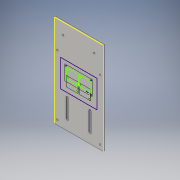
# Autodesk Inventor part: Part2
Saved by Autodesk Inventor 2016 (Build 200138000, 138)
## iProperties
Created: 2015-10-15
Part Number: Part2
Material: Generic
Document SubType Name: Modeling
Designer: hozhu
Density: 1 g/cm^3
Appearance: Default
Author: hozhu
Autodesk Inventor part; units mm, degrees
ref_plane "YZ Plane" through (0, 0, 0) normal (1, 0, 0) x (0, 1, 0)
ref_plane "XZ Plane" through (0, 0, 0) normal (0, 1, 0) x (-1, 0, 0)
ref_plane "XY Plane" through (0, 0, 0) normal (0, 0, 1) x (1, 0, 0)
sketch "Sketch1" plane through (0, 0, 0) normal (0, 0, 1) x (1, 0, 0)
  line L0 (-68.58, -128.7145) -> (68.58, -128.7145)
  line L1 (68.58, -128.7145) -> (68.58, 128.7145)
  line L2 (68.58, 128.7145) -> (-68.58, 128.7145)
  line L3 (-68.58, 128.7145) -> (-68.58, -128.7145)
  line L4 (-68.58, -128.7145) -> (68.58, 128.7145) construction
  line L5 (68.58, -128.7145) -> (-68.58, 128.7145) construction
  point P0 (0, 0)
  dimension "d0" = 137.16
  dimension "d1" = 257.429
  constraints: 12 end point, 2 midpoint, 2 parallel, 1 horizontal, 1 perpendicular
  measures "d0" distance of L1.end L2.end
  measures "d1" distance of L2.end L0.start
extrude "Extrusion1" add sketch "Sketch1" against normal blind 3.175
sketch "Sketch2" plane through (0, 0, 0) normal (0, 0, 1) x (1, 0, 0)
  circle A0 centre (-59.69, 52.5145) radius 2.0955
  line L0 (-68.58, 128.7145) -> (-68.58, -128.7145) projected
  line L1 (-68.58, 128.7145) -> (68.58, 128.7145) projected
  circle A1 centre (59.69, 52.5145) radius 2.0955
  line L2 (68.58, -128.7145) -> (68.58, 128.7145) projected
  circle A2 centre (-59.69, -116.0145) radius 2.0955
  circle A3 centre (59.69, -116.0145) radius 2.0955
  line L3 (-68.58, -128.7145) -> (68.58, -128.7145) projected
  point P0 (0, 0)
  dimension "d4" = 8.89
  dimension "d5" = 76.2
  dimension "d6" = 76.2
  dimension "d7" = 8.89
  dimension "d8" = 4.191
  dimension "d9" = 12.7
  dimension "d10" = 8.89
  dimension "d11" = 8.89
  dimension "d12" = 12.7
  dimension "d13" = 4.191
  dimension "d21" = 4.191
  dimension "d22" = 4.191
  constraints: 4 centre point
  measures "d4" distance from line of L0 A0.centre
  measures "d5" distance from line of L1 A0.centre
  measures "d6" distance from line of L1 A1.centre
  measures "d7" distance from line of A1.centre L2
  measures "d8" diameter of A1
  measures "d9" distance from line of L3 A2.centre
  measures "d10" distance from line of L0 A2.centre
  measures "d11" distance from line of L2 A3.centre
  measures "d12" distance from line of L3 A3.centre
  measures "d13" diameter of A0
  measures "d21" diameter of A2
  measures "d22" diameter of A3
hole "Hole1" at (-59.69, 52.5145, 0) at (59.69, 52.5145, 0) at (-59.69, -116.0145, 0) at (59.69, -116.0145, 0) direction (0, 0, -1) diameter 4.191 end through all
sketch "Sketch4" plane through (0, 0, 0) normal (0, 0, 1) x (1, 0, 0)
  line L0 (-35.179, -49.0855) -> (-35.179, -99.8855)
  line L1 (-28.321, -49.0855) -> (-28.321, -99.8855)
  line L2 (28.321, -49.0855) -> (28.321, -99.8855)
  line L3 (35.179, -49.0855) -> (35.179, -99.8855)
  line L4 (-68.58, 128.7145) -> (-68.58, -128.7145) projected
  line L5 (68.58, -128.7145) -> (68.58, 128.7145) projected
  line L6 (-68.58, -128.7145) -> (68.58, -128.7145) projected
  arc A0 (-28.321, -49.0855) -> (-35.179, -49.0855) centre (-31.75, -49.0855) ccw
  arc A1 (-35.179, -99.8855) -> (-28.321, -99.8855) centre (-31.75, -99.8855) ccw
  arc A2 (35.179, -49.0855) -> (28.321, -49.0855) centre (31.75, -49.0855) ccw
  arc A3 (28.321, -99.8855) -> (35.179, -99.8855) centre (31.75, -99.8855) ccw
  point P0 (0, 0)
  dimension "d23" = 6.858
  dimension "d24" = 6.858
  dimension "d25" = 33.401
  dimension "d26" = 50.8
  dimension "d27" = 33.401
  dimension "d28" = 28.829
  dimension "d29" = 28.829
  dimension "d30" = 28.829
  dimension "d31" = 28.829
  dimension "d32" = 50.8
  dimension "d33" = 50.8
  dimension "d34" = 50.8
  constraints: 8 end point, 8 point on circle, 4 centre point, 4 tangent, 4 vertical
  measures "d23" distance of L1.end L0.end
  measures "d24" distance between parallel lines of L3 L2
  measures "d25" distance between parallel lines of L4 L0
  measures "d26" distance of L3.start L3.end
  measures "d27" distance between parallel lines of L5 L3
  measures "d28" distance from line of L6 L0.end
  measures "d29" distance from line of L6 L1.end
  measures "d30" distance from line of L6 L2.end
  measures "d31" distance from line of L6 L3.end
  measures "d32" distance of L0.start L0.end
  measures "d33" distance of L1.start L1.end
  measures "d34" distance of L2.start L2.end
extrude "Extrusion2" cut sketch "Sketch4" against normal blind 3.175
sketch "Sketch5" plane through (0, 0, 0) normal (0, 0, 1) x (1, 0, 0)
  line L0 (-68.58, 128.7145) -> (68.58, 128.7145) projected
  line L1 (68.58, 128.7145) -> (68.58, -128.7145) projected
  point P0 (0, 0)
  point P1 (-43.3324, 96.9645)
  point P2 (43.3324, 96.9645)
  dimension "d37" = 31.75
  dimension "d38" = 86.6648
  dimension "d39" = 31.75
  dimension "d40" = 25.2476
  measures "d37" distance from line of L0 point (-43.332, 96.964)
  measures "d38" distance of point (-43.332, 96.964) point (43.332, 96.964)
  measures "d39" distance from line of L0 point (43.332, 96.964)
  measures "d40" distance from line of L1 point (43.332, 96.964)
hole "Hole2" at (-43.3324, 96.9645, 0) at (43.3324, 96.9645, 0) direction (0, 0, -1) diameter 4.4704 end through all
sketch "battery_buzzer" plane through (0, 0, 0) normal (0, 0, 1) x (1, 0, 0)
  line L0 (-50.8, 39.8145) -> (50.8, 39.8145)
  line L1 (50.8, 39.8145) -> (50.8, -36.3855)
  line L2 (50.8, -36.3855) -> (-50.8, -36.3855)
  line L3 (-50.8, -36.3855) -> (-50.8, 39.8145)
  line L4 (68.58, -128.7145) -> (68.58, 128.7145) projected
  line L5 (68.58, 128.7145) -> (-68.58, 128.7145) projected
  line L6 (-68.58, 128.7145) -> (-68.58, -128.7145) projected
  line L7 (-34.6353, 23.4567) -> (-1.6153, 23.4567)
  line L8 (-1.6153, 23.4567) -> (-1.6153, -4.4833)
  line L9 (-1.6153, -4.4833) -> (-34.6353, -4.4833)
  line L10 (-34.6353, -4.4833) -> (-34.6353, 23.4567)
  circle A0 centre (-30.8253, 19.6467) radius 1.651
  circle A1 centre (-30.8253, -1.3083) radius 1.651
  circle A2 centre (-5.4253, -1.3083) radius 1.651
  line L11 (0.9247, 23.4567) -> (33.9447, 23.4567)
  line L12 (33.9447, 23.4567) -> (33.9447, -4.4833)
  line L13 (33.9447, -4.4833) -> (0.9247, -4.4833)
  line L14 (0.9247, -4.4833) -> (0.9247, 23.4567)
  circle A3 centre (4.7347, 19.6467) radius 1.651
  circle A4 centre (4.7347, -1.3083) radius 1.651
  circle A5 centre (30.1347, -1.3083) radius 1.651
  point P0 (-1.6153, -4.4833)
  point P1 (48.3688, -4.4833)
  dimension "d48" = 17.78
  dimension "d49" = 88.9
  dimension "d50" = 76.2
  dimension "d51" = 17.78
  dimension "d52" = 33.02
  dimension "d54" = 3.302
  dimension "d55" = 3.302
  dimension "d57" = 3.81
  dimension "d58" = 3.81
  dimension "d59" = 3.81
  dimension "d60" = 20.955
  dimension "d62" = 25.4
  dimension "d74" = 33.02
  dimension "d75" = 3.302
  dimension "d76" = 3.302
  dimension "d77" = 3.81
  dimension "d78" = 3.81
  dimension "d79" = 3.81
  dimension "d80" = 20.955
  dimension "d81" = 25.4
  dimension "d82" = 2.54
  constraints: 24 end point, 7 perpendicular, 6 centre point, 3 horizontal, 2 parallel
  measures "d48" distance between parallel lines of L4 L1
  measures "d49" distance between parallel lines of L5 L0
  measures "d50" distance of L0.end L1.end
  measures "d51" distance between parallel lines of L6 L3
  measures "d52" distance of L7.start L7.end
  measures "d54" diameter of A0
  measures "d55" diameter of A1
  measures "d57" distance from line of L7 A0.centre
  measures "d58" distance from line of L10 A1.centre
  measures "d59" distance from line of L10 A0.centre
  measures "d60" distance of A1.centre A0.centre
  measures "d62" distance of A1.centre A2.centre
  measures "d74" distance of L11.start L12.start
  measures "d75" diameter of A3
  measures "d76" diameter of A4
  measures "d77" distance from line of L11 A3.centre
  measures "d78" distance from line of L14 A4.centre
  measures "d79" distance from line of L14 A3.centre
  measures "d80" distance of A4.centre A3.centre
  measures "d81" distance of A4.centre A5.centre
  measures "d82" distance between parallel lines of L8 L14
sketch "grizzly_bear" plane through (0, 0, 0) normal (0, 0, 1) x (1, 0, 0)
  line L0 (-38.7334, -11.4177) -> (37.4666, -11.4177)
  line L1 (37.4666, -11.4177) -> (37.4666, 29.8573)
  line L2 (37.4666, 29.8573) -> (-38.7334, 29.8573)
  line L3 (-38.7334, 29.8573) -> (-38.7334, -11.4177)
  circle A0 centre (-35.6854, 26.6823) radius 1.651
  circle A1 centre (34.6726, -8.6237) radius 1.651
  circle A2 centre (34.6726, 26.6823) radius 1.651
  circle A3 centre (26.0776, -6.3977) radius 0.45
  circle A4 centre (21.6776, -6.3977) radius 0.45
  point P0 (0, 0)
  dimension "d83" = 3.302
  dimension "d84" = 0.9
  dimension "d85" = 76.2
  dimension "d86" = 41.275
  dimension "d87" = 37.4666
  dimension "d88" = 29.8573
  dimension "d89" = 2.794
  dimension "d90" = 3.175
  dimension "d91" = 2.794
  dimension "d92" = 38.481
  dimension "d93" = 11.389
  dimension "d94" = 36.255
  dimension "d95" = 15.789
  dimension "d96" = 36.255
  dimension "d97" = 73.152
  dimension "d98" = 3.175
  constraints: 8 end point, 5 centre point, 3 equal radius, 2 parallel, 1 horizontal, 1 vertical
  measures "d83" diameter of A2
  measures "d84" diameter of A3
  measures "d85" distance between parallel lines of L1 L3
  measures "d86" distance between parallel lines of L2 L0
  measures "d87" distance from line of point (0, 0) L1
  measures "d88" distance from line of point (0, 0) L2
  measures "d89" distance from line of A2.centre L1
  measures "d90" distance from line of A2.centre L2
  measures "d91" distance from line of A1.centre L1
  measures "d92" distance from line of A1.centre L2
  measures "d93" distance from line of A3.centre L1
  measures "d94" distance from line of A3.centre L2
  measures "d95" distance from line of A4.centre L1
  measures "d96" distance from line of A4.centre L2
  measures "d97" distance from line of A0.centre L1
  measures "d98" distance from line of A0.centre L2
sketch "Smartsensor" plane through (0, 0, 0) normal (0, 0, 1) x (1, 0, 0)
  line L0 (-34.6866, -23.8471) -> (-34.6866, 4.0929)
  line L1 (-34.6866, 4.0929) -> (-1.6666, 4.0929)
  line L2 (-1.6666, 4.0929) -> (-1.6666, -23.8471)
  line L3 (-34.6866, -23.8471) -> (-1.6666, -23.8471)
  circle A0 centre (-30.8766, 0.2829) radius 1.651
  circle A1 centre (-5.4766, -20.6721) radius 1.651
  circle A2 centre (-4.2066, -16.2271) radius 1
  circle A3 centre (-4.2066, -13.6871) radius 1
  circle A4 centre (-4.2066, -11.1471) radius 1
  circle A5 centre (-4.2066, -8.6071) radius 1
  circle A6 centre (-4.2066, -6.0671) radius 1
  circle A7 centre (-4.2066, -3.5271) radius 1
  line L4 (0.8734, -23.8471) -> (0.8734, 4.0929)
  line L5 (0.8734, 4.0929) -> (33.8934, 4.0929)
  line L6 (33.8934, 4.0929) -> (33.8934, -23.8471)
  line L7 (0.8734, -23.8471) -> (33.8934, -23.8471)
  circle A8 centre (4.6834, 0.2829) radius 1.651
  circle A9 centre (30.0834, -20.6721) radius 1.651
  circle A10 centre (31.3534, -16.2271) radius 1
  circle A11 centre (31.3534, -13.6871) radius 1
  circle A12 centre (31.3534, -11.1471) radius 1
  circle A13 centre (31.3534, -8.6071) radius 1
  circle A14 centre (31.3534, -6.0671) radius 1
  circle A15 centre (31.3534, -3.5271) radius 1
  point P0 (0, 0)
  constraints: 16 centre point, 16 end point
body "Solid1"
